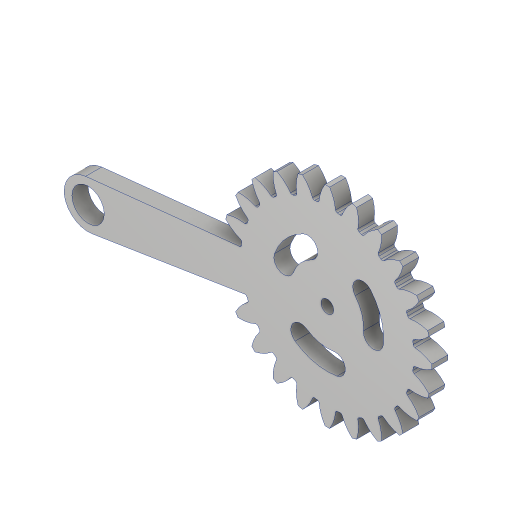
# Autodesk Inventor part: Gear(PCD 48, MOD 2)
Saved by Autodesk Inventor 2023.2 (Build 272271000, 271)
## iProperties
Created: 2021-07-28
Part Number: Gear(PCD 48, MOD 2)
Material: 알루미늄 6061
Document SubType Name: Modeling
Designer: user
Density: 2.7 g/cm^3
Appearance: 알루미늄 - 평지
Mass: 26.9214 g
Surface Area: 65.457 cm^2
Volume: 9.97089 cm^3
Author: user
Autodesk Inventor part; units mm, degrees
(part 1 of 2)
ref_plane "YZ Plane" through (0, 0, 0) normal (1, 0, 0) x (0, 1, 0)
ref_plane "XZ Plane" through (0, 0, 0) normal (0, 1, 0) x (-1, 0, 0)
ref_plane "XY Plane" through (0, 0, 0) normal (0, 0, 1) x (1, 0, 0)
sketch "스케치1" plane through (0, 0, 0) normal (0, 0, 1) x (1, 0, 0)
  arc A0 (1.57, 23.9486) -> (-1.57, 23.9486) centre (0, 0) ccw
  arc A1 (-2.07, 21.4001) -> (2.07, 21.4001) centre (0, 0) ccw
  line L0 (0, 0) -> (0, 26)
  line L1 (-1.57, 0) -> (-1.57, 23.9486)
  line L2 (-0.57, 0) -> (-0.57, 25.9938)
  line L3 (-2.07, 0) -> (-2.07, 21.4001)
  arc A2 (-0.57, 25.9938) -> (-2.07, 21.4001) centre (7.2779, 20.8894) ccw
  line L4 (1.57, 0) -> (1.57, 23.9486)
  line L5 (0.57, 0) -> (0.57, 25.9938)
  line L6 (2.07, 0) -> (2.07, 21.4001)
  arc A3 (2.07, 21.4001) -> (0.57, 25.9938) centre (-7.2779, 20.8894) ccw
  arc A4 (0.57, 25.9938) -> (-0.57, 25.9938) centre (0, 0) ccw
  point P0 (-1.57, 29)
  point P1 (-0.57, 29)
  point P2 (-2.07, 29)
  point P3 (1.57, 29)
  point P4 (0.57, 29)
  point P5 (2.07, 29)
  dimension "d0" = 48
  dimension "d2" = 43
  dimension "d3" = 1.57
  dimension "d4" = 1
  dimension "d7" = 0.5
  constraints: 14 end point, 13 point on circle, 9 symmetric about line, 5 centre point, 3 coincident, 3 parallel, 1 vertical, 1 other
  measures "d0" diameter of A0
  measures "d2" diameter of A1
  measures "d3" distance between parallel lines of L0 L1
  measures "d4" distance between parallel lines of L1 L2
  measures "d7" distance between parallel lines of L3 L1
extrude "돌출1" add sketch "스케치1" along normal blind 4
sketch "스케치11" plane through (0, 0, 4) normal (0, 0, 1) x (1, 0, 0)
  circle A0 centre (0, 0) radius 1.6 projected
  arc A1 (13.9479, -1.2066) -> (10.7334, 8.9886) centre (0, 0) ccw projected
  arc A2 (8.9665, -0.7757) -> (13.9479, -1.2066) centre (11.4572, -0.9911) ccw projected
  arc A3 (8.9665, -0.7757) -> (6.9, 5.7784) centre (0, 0) ccw projected
  arc A4 (10.7334, 8.9886) -> (6.9, 5.7784) centre (8.8167, 7.3835) ccw projected
  arc A5 (-8.0189, -11.476) -> (2.4176, -13.7897) centre (0, 0) ccw projected
  arc A6 (-5.155, -7.3774) -> (-8.0189, -11.476) centre (-6.5869, -9.4267) ccw projected
  arc A7 (-5.155, -7.3774) -> (1.5542, -8.8648) centre (0, 0) ccw projected
  arc A8 (2.4176, -13.7897) -> (1.5542, -8.8648) centre (1.9859, -11.3272) ccw projected
  arc A9 (-3.8115, 8.1531) -> (-8.4542, 3.0864) centre (0, 0) ccw projected
  arc A10 (-13.151, 4.8011) -> (-8.4542, 3.0864) centre (-10.8026, 3.9438) ccw projected
  arc A11 (-5.929, 12.6825) -> (-13.151, 4.8011) centre (0, 0) ccw projected
  arc A12 (-3.8115, 8.1531) -> (-5.929, 12.6825) centre (-4.8703, 10.4178) ccw projected
  circle A13 centre (-59.4867, -7.8316) radius 4.025 projected
  arc A14 (-60.1049, -2.02) -> (-65.4557, -8.4603) centre (-59.4744, -7.9868) ccw projected
  arc A15 (-65.4557, -8.4603) -> (-58.5717, -13.6038) centre (-59.507, -7.6772) ccw projected
  line L0 (-58.5717, -13.6038) -> (-20.5345, -7.6012) projected
  arc A16 (-19.9916, -7.9111) -> (-20.5345, -7.6012) centre (-20.4565, -8.0951) ccw projected
  arc A17 (-19.9916, -7.9111) -> (-19.7349, -8.5314) centre (0, 0) ccw projected
  arc A18 (-19.9027, -9.1363) -> (-19.7349, -8.5314) centre (-20.1938, -8.7298) ccw projected
  arc A19 (-19.9027, -9.1363) -> (-22.7962, -12.5032) centre (-14.4518, -16.7475) ccw projected
  arc A20 (-22.7962, -12.5032) -> (-22.2262, -13.4905) centre (0, 0) ccw projected
  arc A21 (-22.2262, -13.4905) -> (-17.8636, -12.6681) centre (-21.7297, -4.1418) ccw projected
  arc A22 (-17.2558, -12.8252) -> (-17.8636, -12.6681) centre (-17.6571, -13.1235) ccw projected
  arc A23 (-17.2558, -12.8252) -> (-16.8544, -13.3484) centre (0, 0) ccw projected
  arc A24 (-16.8599, -13.9762) -> (-16.8544, -13.3484) centre (-17.2463, -13.6589) ccw projected
  arc A25 (-16.8599, -13.9762) -> (-18.7834, -17.9773) centre (-9.6248, -19.9173) ccw projected
  arc A26 (-18.7834, -17.9773) -> (-17.9773, -18.7834) centre (0, 0) ccw projected
  arc A27 (-17.9773, -18.7834) -> (-13.9762, -16.8599) centre (-19.9173, -9.6248) ccw projected
  arc A28 (-13.3484, -16.8544) -> (-13.9762, -16.8599) centre (-13.6589, -17.2463) ccw projected
  arc A29 (-13.3484, -16.8544) -> (-12.8252, -17.2558) centre (0, 0) ccw projected
  arc A30 (-12.6681, -17.8636) -> (-12.8252, -17.2558) centre (-13.1235, -17.6571) ccw projected
  arc A31 (-12.6681, -17.8636) -> (-13.4905, -22.2262) centre (-4.1418, -21.7297) ccw projected
  arc A32 (-13.4905, -22.2262) -> (-12.5032, -22.7962) centre (0, 0) ccw projected
  arc A33 (-12.5032, -22.7962) -> (-9.1363, -19.9027) centre (-16.7475, -14.4518) ccw projected
  arc A34 (-8.5314, -19.7349) -> (-9.1363, -19.9027) centre (-8.7298, -20.1938) ccw projected
  arc A35 (-8.5314, -19.7349) -> (-7.9221, -19.9873) centre (0, 0) ccw projected
  arc A36 (-7.613, -20.5337) -> (-7.9221, -19.9873) centre (-8.1063, -20.4521) ccw projected
  arc A37 (-7.613, -20.5337) -> (-7.2783, -24.9605) centre (1.6233, -22.0613) ccw projected
  arc A38 (-7.2783, -24.9605) -> (-6.1771, -25.2556) centre (0, 0) ccw projected
  arc A39 (-6.1771, -25.2556) -> (-3.6738, -21.5892) centre (-12.4365, -18.2939) ccw projected
  arc A40 (-3.1329, -21.2705) -> (-3.6738, -21.5892) centre (-3.2058, -21.7652) ccw projected
  arc A41 (-3.1329, -21.2705) -> (-2.4791, -21.3566) centre (0, 0) ccw projected
  arc A42 (-2.0391, -21.8044) -> (-2.4791, -21.3566) centre (-2.5367, -21.8533) ccw projected
  arc A43 (-2.0391, -21.8044) -> (-0.57, -25.9938) centre (7.2779, -20.8894) ccw projected
  arc A44 (-0.57, -25.9938) -> (0.57, -25.9938) centre (0, 0) ccw projected
  arc A45 (0.57, -25.9938) -> (2.0391, -21.8044) centre (-7.2779, -20.8894) ccw projected
  arc A46 (2.4791, -21.3566) -> (2.0391, -21.8044) centre (2.5367, -21.8533) ccw projected
  arc A47 (2.4791, -21.3566) -> (3.1329, -21.2705) centre (0, 0) ccw projected
  arc A48 (3.6738, -21.5892) -> (3.1329, -21.2705) centre (3.2058, -21.7652) ccw projected
  arc A49 (3.6738, -21.5892) -> (6.1771, -25.2556) centre (12.4365, -18.2939) ccw projected
  arc A50 (6.1771, -25.2556) -> (7.2783, -24.9605) centre (0, 0) ccw projected
  arc A51 (7.2783, -24.9605) -> (7.613, -20.5337) centre (-1.6233, -22.0613) ccw projected
  arc A52 (7.9221, -19.9873) -> (7.613, -20.5337) centre (8.1063, -20.4521) ccw projected
  arc A53 (7.9221, -19.9873) -> (8.5314, -19.7349) centre (0, 0) ccw projected
  arc A54 (9.1363, -19.9027) -> (8.5314, -19.7349) centre (8.7298, -20.1938) ccw projected
  arc A55 (9.1363, -19.9027) -> (12.5032, -22.7962) centre (16.7475, -14.4518) ccw projected
  arc A56 (12.5032, -22.7962) -> (13.4905, -22.2262) centre (0, 0) ccw projected
  arc A57 (13.4905, -22.2262) -> (12.6681, -17.8636) centre (4.1418, -21.7297) ccw projected
  arc A58 (12.8252, -17.2558) -> (12.6681, -17.8636) centre (13.1235, -17.6571) ccw projected
  arc A59 (12.8252, -17.2558) -> (13.3484, -16.8544) centre (0, 0) ccw projected
  arc A60 (13.9762, -16.8599) -> (13.3484, -16.8544) centre (13.6589, -17.2463) ccw projected
  arc A61 (13.9762, -16.8599) -> (17.9773, -18.7834) centre (19.9173, -9.6248) ccw projected
  arc A62 (17.9773, -18.7834) -> (18.7834, -17.9773) centre (0, 0) ccw projected
  arc A63 (18.7834, -17.9773) -> (16.8599, -13.9762) centre (9.6248, -19.9173) ccw projected
  arc A64 (16.8544, -13.3484) -> (16.8599, -13.9762) centre (17.2463, -13.6589) ccw projected
  arc A65 (16.8544, -13.3484) -> (17.2558, -12.8252) centre (0, 0) ccw projected
  arc A66 (17.8636, -12.6681) -> (17.2558, -12.8252) centre (17.6571, -13.1235) ccw projected
  arc A67 (17.8636, -12.6681) -> (22.2262, -13.4905) centre (21.7297, -4.1418) ccw projected
  arc A68 (22.2262, -13.4905) -> (22.7962, -12.5032) centre (0, 0) ccw projected
  arc A69 (22.7962, -12.5032) -> (19.9027, -9.1363) centre (14.4518, -16.7475) ccw projected
  arc A70 (19.7349, -8.5314) -> (19.9027, -9.1363) centre (20.1938, -8.7298) ccw projected
  arc A71 (19.7349, -8.5314) -> (19.9873, -7.9221) centre (0, 0) ccw projected
  arc A72 (20.5337, -7.613) -> (19.9873, -7.9221) centre (20.4521, -8.1063) ccw projected
  arc A73 (20.5337, -7.613) -> (24.9605, -7.2783) centre (22.0613, 1.6233) ccw projected
  arc A74 (24.9605, -7.2783) -> (25.2556, -6.1771) centre (0, 0) ccw projected
  arc A75 (25.2556, -6.1771) -> (21.5892, -3.6738) centre (18.2939, -12.4365) ccw projected
  arc A76 (21.2705, -3.1329) -> (21.5892, -3.6738) centre (21.7652, -3.2058) ccw projected
  arc A77 (21.2705, -3.1329) -> (21.3566, -2.4791) centre (0, 0) ccw projected
  arc A78 (21.8044, -2.0391) -> (21.3566, -2.4791) centre (21.8533, -2.5367) ccw projected
  arc A79 (21.8044, -2.0391) -> (25.9938, -0.57) centre (20.8894, 7.2779) ccw projected
  arc A80 (25.9938, -0.57) -> (25.9938, 0.57) centre (0, 0) ccw projected
  arc A81 (25.9938, 0.57) -> (21.8044, 2.0391) centre (20.8894, -7.2779) ccw projected
  arc A82 (21.3566, 2.4791) -> (21.8044, 2.0391) centre (21.8533, 2.5367) ccw projected
  arc A83 (21.3566, 2.4791) -> (21.2705, 3.1329) centre (0, 0) ccw projected
  arc A84 (21.5892, 3.6738) -> (21.2705, 3.1329) centre (21.7652, 3.2058) ccw projected
  arc A85 (21.5892, 3.6738) -> (25.2556, 6.1771) centre (18.2939, 12.4365) ccw projected
  arc A86 (25.2556, 6.1771) -> (24.9605, 7.2783) centre (0, 0) ccw projected
  arc A87 (24.9605, 7.2783) -> (20.5337, 7.613) centre (22.0613, -1.6233) ccw projected
  arc A88 (19.9873, 7.9221) -> (20.5337, 7.613) centre (20.4521, 8.1063) ccw projected
  arc A89 (19.9873, 7.9221) -> (19.7349, 8.5314) centre (0, 0) ccw projected
  arc A90 (19.9027, 9.1363) -> (19.7349, 8.5314) centre (20.1938, 8.7298) ccw projected
  arc A91 (19.9027, 9.1363) -> (22.7962, 12.5032) centre (14.4518, 16.7475) ccw projected
  arc A92 (22.7962, 12.5032) -> (22.2262, 13.4905) centre (0, 0) ccw projected
  arc A93 (22.2262, 13.4905) -> (17.8636, 12.6681) centre (21.7297, 4.1418) ccw projected
  arc A94 (17.2558, 12.8252) -> (17.8636, 12.6681) centre (17.6571, 13.1235) ccw projected
  arc A95 (17.2558, 12.8252) -> (16.8544, 13.3484) centre (0, 0) ccw projected
  arc A96 (16.8599, 13.9762) -> (16.8544, 13.3484) centre (17.2463, 13.6589) ccw projected
  arc A97 (16.8599, 13.9762) -> (18.7834, 17.9773) centre (9.6248, 19.9173) ccw projected
  arc A98 (18.7834, 17.9773) -> (17.9773, 18.7834) centre (0, 0) ccw projected
  arc A99 (17.9773, 18.7834) -> (13.9762, 16.8599) centre (19.9173, 9.6248) ccw projected
  arc A100 (13.3484, 16.8544) -> (13.9762, 16.8599) centre (13.6589, 17.2463) ccw projected
  arc A101 (13.3484, 16.8544) -> (12.8252, 17.2558) centre (0, 0) ccw projected
  arc A102 (12.6681, 17.8636) -> (12.8252, 17.2558) centre (13.1235, 17.6571) ccw projected
  arc A103 (12.6681, 17.8636) -> (13.4905, 22.2262) centre (4.1418, 21.7297) ccw projected
  arc A104 (13.4905, 22.2262) -> (12.5032, 22.7962) centre (0, 0) ccw projected
  arc A105 (12.5032, 22.7962) -> (9.1363, 19.9027) centre (16.7475, 14.4518) ccw projected
  arc A106 (8.5314, 19.7349) -> (9.1363, 19.9027) centre (8.7298, 20.1938) ccw projected
  arc A107 (8.5314, 19.7349) -> (7.9221, 19.9873) centre (0, 0) ccw projected
  arc A108 (7.613, 20.5337) -> (7.9221, 19.9873) centre (8.1063, 20.4521) ccw projected
  arc A109 (7.613, 20.5337) -> (7.2783, 24.9605) centre (-1.6233, 22.0613) ccw projected
  arc A110 (7.2783, 24.9605) -> (6.1771, 25.2556) centre (0, 0) ccw projected
  arc A111 (6.1771, 25.2556) -> (3.6738, 21.5892) centre (12.4365, 18.2939) ccw projected
  arc A112 (3.1329, 21.2705) -> (3.6738, 21.5892) centre (3.2058, 21.7652) ccw projected
  arc A113 (3.1329, 21.2705) -> (2.4791, 21.3566) centre (0, 0) ccw projected
  arc A114 (2.0391, 21.8044) -> (2.4791, 21.3566) centre (2.5367, 21.8533) ccw projected
  arc A115 (2.0391, 21.8044) -> (0.57, 25.9938) centre (-7.2779, 20.8894) ccw projected
  arc A116 (0.57, 25.9938) -> (-0.57, 25.9938) centre (0, 0) ccw projected
  arc A117 (-0.57, 25.9938) -> (-2.0391, 21.8044) centre (7.2779, 20.8894) ccw projected
  arc A118 (-2.4791, 21.3566) -> (-2.0391, 21.8044) centre (-2.5367, 21.8533) ccw projected
  arc A119 (-2.4791, 21.3566) -> (-3.1329, 21.2705) centre (0, 0) ccw projected
  arc A120 (-3.6738, 21.5892) -> (-3.1329, 21.2705) centre (-3.2058, 21.7652) ccw projected
  arc A121 (-3.6738, 21.5892) -> (-6.1771, 25.2556) centre (-12.4365, 18.2939) ccw projected
  arc A122 (-6.1771, 25.2556) -> (-7.2783, 24.9605) centre (0, 0) ccw projected
  arc A123 (-7.2783, 24.9605) -> (-7.613, 20.5337) centre (1.6233, 22.0613) ccw projected
  arc A124 (-7.9221, 19.9873) -> (-7.613, 20.5337) centre (-8.1063, 20.4521) ccw projected
  arc A125 (-7.9221, 19.9873) -> (-8.5314, 19.7349) centre (0, 0) ccw projected
  arc A126 (-9.1363, 19.9027) -> (-8.5314, 19.7349) centre (-8.7298, 20.1938) ccw projected
  arc A127 (-9.1363, 19.9027) -> (-12.5032, 22.7962) centre (-16.7475, 14.4518) ccw projected
  arc A128 (-12.5032, 22.7962) -> (-13.4905, 22.2262) centre (0, 0) ccw projected
  arc A129 (-13.4905, 22.2262) -> (-12.6681, 17.8636) centre (-4.1418, 21.7297) ccw projected
  arc A130 (-12.8252, 17.2558) -> (-12.6681, 17.8636) centre (-13.1235, 17.6571) ccw projected
  arc A131 (-12.8252, 17.2558) -> (-13.3484, 16.8544) centre (0, 0) ccw projected
  arc A132 (-13.9762, 16.8599) -> (-13.3484, 16.8544) centre (-13.6589, 17.2463) ccw projected
  arc A133 (-13.9762, 16.8599) -> (-17.9773, 18.7834) centre (-19.9173, 9.6248) ccw projected
  arc A134 (-17.9773, 18.7834) -> (-18.7834, 17.9773) centre (0, 0) ccw projected
  arc A135 (-18.7834, 17.9773) -> (-16.8599, 13.9762) centre (-9.6248, 19.9173) ccw projected
  arc A136 (-16.8544, 13.3484) -> (-16.8599, 13.9762) centre (-17.2463, 13.6589) ccw projected
  arc A137 (-16.8544, 13.3484) -> (-17.2558, 12.8252) centre (0, 0) ccw projected
  arc A138 (-17.8636, 12.6681) -> (-17.2558, 12.8252) centre (-17.6571, 13.1235) ccw projected
  arc A139 (-17.8636, 12.6681) -> (-22.2262, 13.4905) centre (-21.7297, 4.1418) ccw projected
  arc A140 (-22.2262, 13.4905) -> (-22.7962, 12.5032) centre (0, 0) ccw projected
  arc A141 (-22.7962, 12.5032) -> (-19.9027, 9.1363) centre (-14.4518, 16.7475) ccw projected
  arc A142 (-19.7349, 8.5314) -> (-19.9027, 9.1363) centre (-20.1938, 8.7298) ccw projected
  arc A143 (-19.7349, 8.5314) -> (-19.9873, 7.9221) centre (0, 0) ccw projected
  arc A144 (-20.5337, 7.613) -> (-19.9873, 7.9221) centre (-20.4521, 8.1063) ccw projected
  arc A145 (-20.5337, 7.613) -> (-24.9605, 7.2783) centre (-22.0613, -1.6233) ccw projected
  arc A146 (-24.9605, 7.2783) -> (-25.2556, 6.1771) centre (0, 0) ccw projected
  arc A147 (-25.2556, 6.1771) -> (-21.5892, 3.6738) centre (-18.2939, 12.4365) ccw projected
  arc A148 (-21.2705, 3.1329) -> (-21.5892, 3.6738) centre (-21.7652, 3.2058) ccw projected
  arc A149 (-21.2705, 3.1329) -> (-21.358, 2.4674) centre (0, 0) ccw projected
  arc A150 (-21.8021, 2.0275) -> (-21.358, 2.4674) centre (-21.8546, 2.5248) ccw projected
  line L1 (-21.8021, 2.0275) -> (-60.1049, -2.02) projected
  circle A151 centre (0, 0) radius 1.6 projected
  circle A152 centre (0, 0) radius 1.6
  constraints: 1 centre point, 1 coincident
sketch "스케치7" plane through (0, 0, 4) normal (0, 0, 1) x (1, 0, 0)
  circle A0 centre (-59.4867, -7.8316) radius 4.025 projected
  circle A1 centre (-59.4867, -7.8316) radius 4.8
  point P0 (0, 0)
  dimension "d46" = 9.6
  constraints: 1 centre point, 1 coincident
  measures "d46" diameter of A1
sketch "스케치8" plane through (0, 0, 4) normal (0, 0, 1) x (1, 0, 0)
  circle A0 centre (-59.4867, -7.8316) radius 4.8 projected
  arc A1 (13.9479, -1.2066) -> (10.7334, 8.9886) centre (0, 0) ccw projected
  arc A2 (8.9665, -0.7757) -> (13.9479, -1.2066) centre (11.4572, -0.9911) ccw projected
  arc A3 (8.9665, -0.7757) -> (6.9, 5.7784) centre (0, 0) ccw projected
  arc A4 (10.7334, 8.9886) -> (6.9, 5.7784) centre (8.8167, 7.3835) ccw projected
  arc A5 (-8.0189, -11.476) -> (2.4176, -13.7897) centre (0, 0) ccw projected
  arc A6 (-5.155, -7.3774) -> (-8.0189, -11.476) centre (-6.5869, -9.4267) ccw projected
  arc A7 (-5.155, -7.3774) -> (1.5542, -8.8648) centre (0, 0) ccw projected
  arc A8 (2.4176, -13.7897) -> (1.5542, -8.8648) centre (1.9859, -11.3272) ccw projected
  arc A9 (-3.8115, 8.1531) -> (-8.4542, 3.0864) centre (0, 0) ccw projected
  arc A10 (-13.151, 4.8011) -> (-8.4542, 3.0864) centre (-10.8026, 3.9438) ccw projected
  arc A11 (-5.929, 12.6825) -> (-13.151, 4.8011) centre (0, 0) ccw projected
  arc A12 (-3.8115, 8.1531) -> (-5.929, 12.6825) centre (-4.8703, 10.4178) ccw projected
  arc A13 (-60.1049, -2.02) -> (-65.4557, -8.4603) centre (-59.4744, -7.9868) ccw projected
  arc A14 (-65.4557, -8.4603) -> (-58.5717, -13.6038) centre (-59.507, -7.6772) ccw projected
  line L0 (-58.5717, -13.6038) -> (-20.5345, -7.6012) projected
  arc A15 (-19.9916, -7.9111) -> (-20.5345, -7.6012) centre (-20.4565, -8.0951) ccw projected
  arc A16 (-19.9916, -7.9111) -> (-19.7349, -8.5314) centre (0, 0) ccw projected
  arc A17 (-19.9027, -9.1363) -> (-19.7349, -8.5314) centre (-20.1938, -8.7298) ccw projected
  arc A18 (-19.9027, -9.1363) -> (-22.7962, -12.5032) centre (-14.4518, -16.7475) ccw projected
  arc A19 (-22.7962, -12.5032) -> (-22.2262, -13.4905) centre (0, 0) ccw projected
  arc A20 (-22.2262, -13.4905) -> (-17.8636, -12.6681) centre (-21.7297, -4.1418) ccw projected
  arc A21 (-17.2558, -12.8252) -> (-17.8636, -12.6681) centre (-17.6571, -13.1235) ccw projected
  arc A22 (-17.2558, -12.8252) -> (-16.8544, -13.3484) centre (0, 0) ccw projected
  arc A23 (-16.8599, -13.9762) -> (-16.8544, -13.3484) centre (-17.2463, -13.6589) ccw projected
  arc A24 (-16.8599, -13.9762) -> (-18.7834, -17.9773) centre (-9.6248, -19.9173) ccw projected
  arc A25 (-18.7834, -17.9773) -> (-17.9773, -18.7834) centre (0, 0) ccw projected
  arc A26 (-17.9773, -18.7834) -> (-13.9762, -16.8599) centre (-19.9173, -9.6248) ccw projected
  arc A27 (-13.3484, -16.8544) -> (-13.9762, -16.8599) centre (-13.6589, -17.2463) ccw projected
  arc A28 (-13.3484, -16.8544) -> (-12.8252, -17.2558) centre (0, 0) ccw projected
  arc A29 (-12.6681, -17.8636) -> (-12.8252, -17.2558) centre (-13.1235, -17.6571) ccw projected
  arc A30 (-12.6681, -17.8636) -> (-13.4905, -22.2262) centre (-4.1418, -21.7297) ccw projected
  arc A31 (-13.4905, -22.2262) -> (-12.5032, -22.7962) centre (0, 0) ccw projected
  arc A32 (-12.5032, -22.7962) -> (-9.1363, -19.9027) centre (-16.7475, -14.4518) ccw projected
  arc A33 (-8.5314, -19.7349) -> (-9.1363, -19.9027) centre (-8.7298, -20.1938) ccw projected
  arc A34 (-8.5314, -19.7349) -> (-7.9221, -19.9873) centre (0, 0) ccw projected
  arc A35 (-7.613, -20.5337) -> (-7.9221, -19.9873) centre (-8.1063, -20.4521) ccw projected
  arc A36 (-7.613, -20.5337) -> (-7.2783, -24.9605) centre (1.6233, -22.0613) ccw projected
  arc A37 (-7.2783, -24.9605) -> (-6.1771, -25.2556) centre (0, 0) ccw projected
  arc A38 (-6.1771, -25.2556) -> (-3.6738, -21.5892) centre (-12.4365, -18.2939) ccw projected
  arc A39 (-3.1329, -21.2705) -> (-3.6738, -21.5892) centre (-3.2058, -21.7652) ccw projected
  arc A40 (-3.1329, -21.2705) -> (-2.4791, -21.3566) centre (0, 0) ccw projected
  arc A41 (-2.0391, -21.8044) -> (-2.4791, -21.3566) centre (-2.5367, -21.8533) ccw projected
  arc A42 (-2.0391, -21.8044) -> (-0.57, -25.9938) centre (7.2779, -20.8894) ccw projected
  arc A43 (-0.57, -25.9938) -> (0.57, -25.9938) centre (0, 0) ccw projected
  arc A44 (0.57, -25.9938) -> (2.0391, -21.8044) centre (-7.2779, -20.8894) ccw projected
  arc A45 (2.4791, -21.3566) -> (2.0391, -21.8044) centre (2.5367, -21.8533) ccw projected
  arc A46 (2.4791, -21.3566) -> (3.1329, -21.2705) centre (0, 0) ccw projected
  arc A47 (3.6738, -21.5892) -> (3.1329, -21.2705) centre (3.2058, -21.7652) ccw projected
  arc A48 (3.6738, -21.5892) -> (6.1771, -25.2556) centre (12.4365, -18.2939) ccw projected
  arc A49 (6.1771, -25.2556) -> (7.2783, -24.9605) centre (0, 0) ccw projected
  arc A50 (7.2783, -24.9605) -> (7.613, -20.5337) centre (-1.6233, -22.0613) ccw projected
  arc A51 (7.9221, -19.9873) -> (7.613, -20.5337) centre (8.1063, -20.4521) ccw projected
  arc A52 (7.9221, -19.9873) -> (8.5314, -19.7349) centre (0, 0) ccw projected
  arc A53 (9.1363, -19.9027) -> (8.5314, -19.7349) centre (8.7298, -20.1938) ccw projected
  arc A54 (9.1363, -19.9027) -> (12.5032, -22.7962) centre (16.7475, -14.4518) ccw projected
  arc A55 (12.5032, -22.7962) -> (13.4905, -22.2262) centre (0, 0) ccw projected
  arc A56 (13.4905, -22.2262) -> (12.6681, -17.8636) centre (4.1418, -21.7297) ccw projected
  arc A57 (12.8252, -17.2558) -> (12.6681, -17.8636) centre (13.1235, -17.6571) ccw projected
  arc A58 (12.8252, -17.2558) -> (13.3484, -16.8544) centre (0, 0) ccw projected
  arc A59 (13.9762, -16.8599) -> (13.3484, -16.8544) centre (13.6589, -17.2463) ccw projected
  arc A60 (13.9762, -16.8599) -> (17.9773, -18.7834) centre (19.9173, -9.6248) ccw projected
  arc A61 (17.9773, -18.7834) -> (18.7834, -17.9773) centre (0, 0) ccw projected
  arc A62 (18.7834, -17.9773) -> (16.8599, -13.9762) centre (9.6248, -19.9173) ccw projected
  arc A63 (16.8544, -13.3484) -> (16.8599, -13.9762) centre (17.2463, -13.6589) ccw projected
  arc A64 (16.8544, -13.3484) -> (17.2558, -12.8252) centre (0, 0) ccw projected
  arc A65 (17.8636, -12.6681) -> (17.2558, -12.8252) centre (17.6571, -13.1235) ccw projected
  arc A66 (17.8636, -12.6681) -> (22.2262, -13.4905) centre (21.7297, -4.1418) ccw projected
  arc A67 (22.2262, -13.4905) -> (22.7962, -12.5032) centre (0, 0) ccw projected
  arc A68 (22.7962, -12.5032) -> (19.9027, -9.1363) centre (14.4518, -16.7475) ccw projected
  arc A69 (19.7349, -8.5314) -> (19.9027, -9.1363) centre (20.1938, -8.7298) ccw projected
  arc A70 (19.7349, -8.5314) -> (19.9873, -7.9221) centre (0, 0) ccw projected
  arc A71 (20.5337, -7.613) -> (19.9873, -7.9221) centre (20.4521, -8.1063) ccw projected
  arc A72 (20.5337, -7.613) -> (24.9605, -7.2783) centre (22.0613, 1.6233) ccw projected
  arc A73 (24.9605, -7.2783) -> (25.2556, -6.1771) centre (0, 0) ccw projected
  arc A74 (25.2556, -6.1771) -> (21.5892, -3.6738) centre (18.2939, -12.4365) ccw projected
  arc A75 (21.2705, -3.1329) -> (21.5892, -3.6738) centre (21.7652, -3.2058) ccw projected
  arc A76 (21.2705, -3.1329) -> (21.3566, -2.4791) centre (0, 0) ccw projected
  arc A77 (21.8044, -2.0391) -> (21.3566, -2.4791) centre (21.8533, -2.5367) ccw projected
  arc A78 (21.8044, -2.0391) -> (25.9938, -0.57) centre (20.8894, 7.2779) ccw projected
  arc A79 (25.9938, -0.57) -> (25.9938, 0.57) centre (0, 0) ccw projected
  arc A80 (25.9938, 0.57) -> (21.8044, 2.0391) centre (20.8894, -7.2779) ccw projected
  arc A81 (21.3566, 2.4791) -> (21.8044, 2.0391) centre (21.8533, 2.5367) ccw projected
  arc A82 (21.3566, 2.4791) -> (21.2705, 3.1329) centre (0, 0) ccw projected
  arc A83 (21.5892, 3.6738) -> (21.2705, 3.1329) centre (21.7652, 3.2058) ccw projected
  arc A84 (21.5892, 3.6738) -> (25.2556, 6.1771) centre (18.2939, 12.4365) ccw projected
  arc A85 (25.2556, 6.1771) -> (24.9605, 7.2783) centre (0, 0) ccw projected
  arc A86 (24.9605, 7.2783) -> (20.5337, 7.613) centre (22.0613, -1.6233) ccw projected
  arc A87 (19.9873, 7.9221) -> (20.5337, 7.613) centre (20.4521, 8.1063) ccw projected
  arc A88 (19.9873, 7.9221) -> (19.7349, 8.5314) centre (0, 0) ccw projected
  arc A89 (19.9027, 9.1363) -> (19.7349, 8.5314) centre (20.1938, 8.7298) ccw projected
  arc A90 (19.9027, 9.1363) -> (22.7962, 12.5032) centre (14.4518, 16.7475) ccw projected
  arc A91 (22.7962, 12.5032) -> (22.2262, 13.4905) centre (0, 0) ccw projected
  arc A92 (22.2262, 13.4905) -> (17.8636, 12.6681) centre (21.7297, 4.1418) ccw projected
  arc A93 (17.2558, 12.8252) -> (17.8636, 12.6681) centre (17.6571, 13.1235) ccw projected
  arc A94 (17.2558, 12.8252) -> (16.8544, 13.3484) centre (0, 0) ccw projected
  arc A95 (16.8599, 13.9762) -> (16.8544, 13.3484) centre (17.2463, 13.6589) ccw projected
  arc A96 (16.8599, 13.9762) -> (18.7834, 17.9773) centre (9.6248, 19.9173) ccw projected
  arc A97 (18.7834, 17.9773) -> (17.9773, 18.7834) centre (0, 0) ccw projected
  arc A98 (17.9773, 18.7834) -> (13.9762, 16.8599) centre (19.9173, 9.6248) ccw projected
  arc A99 (13.3484, 16.8544) -> (13.9762, 16.8599) centre (13.6589, 17.2463) ccw projected
  arc A100 (13.3484, 16.8544) -> (12.8252, 17.2558) centre (0, 0) ccw projected
  arc A101 (12.6681, 17.8636) -> (12.8252, 17.2558) centre (13.1235, 17.6571) ccw projected
  arc A102 (12.6681, 17.8636) -> (13.4905, 22.2262) centre (4.1418, 21.7297) ccw projected
  arc A103 (13.4905, 22.2262) -> (12.5032, 22.7962) centre (0, 0) ccw projected
  arc A104 (12.5032, 22.7962) -> (9.1363, 19.9027) centre (16.7475, 14.4518) ccw projected
  arc A105 (8.5314, 19.7349) -> (9.1363, 19.9027) centre (8.7298, 20.1938) ccw projected
  arc A106 (8.5314, 19.7349) -> (7.9221, 19.9873) centre (0, 0) ccw projected
  arc A107 (7.613, 20.5337) -> (7.9221, 19.9873) centre (8.1063, 20.4521) ccw projected
  arc A108 (7.613, 20.5337) -> (7.2783, 24.9605) centre (-1.6233, 22.0613) ccw projected
  arc A109 (7.2783, 24.9605) -> (6.1771, 25.2556) centre (0, 0) ccw projected
  arc A110 (6.1771, 25.2556) -> (3.6738, 21.5892) centre (12.4365, 18.2939) ccw projected
  arc A111 (3.1329, 21.2705) -> (3.6738, 21.5892) centre (3.2058, 21.7652) ccw projected
  arc A112 (3.1329, 21.2705) -> (2.4791, 21.3566) centre (0, 0) ccw projected
  arc A113 (2.0391, 21.8044) -> (2.4791, 21.3566) centre (2.5367, 21.8533) ccw projected
  arc A114 (2.0391, 21.8044) -> (0.57, 25.9938) centre (-7.2779, 20.8894) ccw projected
  arc A115 (0.57, 25.9938) -> (-0.57, 25.9938) centre (0, 0) ccw projected
  arc A116 (-0.57, 25.9938) -> (-2.0391, 21.8044) centre (7.2779, 20.8894) ccw projected
  arc A117 (-2.4791, 21.3566) -> (-2.0391, 21.8044) centre (-2.5367, 21.8533) ccw projected
  arc A118 (-2.4791, 21.3566) -> (-3.1329, 21.2705) centre (0, 0) ccw projected
  arc A119 (-3.6738, 21.5892) -> (-3.1329, 21.2705) centre (-3.2058, 21.7652) ccw projected
  arc A120 (-3.6738, 21.5892) -> (-6.1771, 25.2556) centre (-12.4365, 18.2939) ccw projected
  arc A121 (-6.1771, 25.2556) -> (-7.2783, 24.9605) centre (0, 0) ccw projected
  arc A122 (-7.2783, 24.9605) -> (-7.613, 20.5337) centre (1.6233, 22.0613) ccw projected
  arc A123 (-7.9221, 19.9873) -> (-7.613, 20.5337) centre (-8.1063, 20.4521) ccw projected
  arc A124 (-7.9221, 19.9873) -> (-8.5314, 19.7349) centre (0, 0) ccw projected
  arc A125 (-9.1363, 19.9027) -> (-8.5314, 19.7349) centre (-8.7298, 20.1938) ccw projected
  arc A126 (-9.1363, 19.9027) -> (-12.5032, 22.7962) centre (-16.7475, 14.4518) ccw projected
  arc A127 (-12.5032, 22.7962) -> (-13.4905, 22.2262) centre (0, 0) ccw projected
  arc A128 (-13.4905, 22.2262) -> (-12.6681, 17.8636) centre (-4.1418, 21.7297) ccw projected
  arc A129 (-12.8252, 17.2558) -> (-12.6681, 17.8636) centre (-13.1235, 17.6571) ccw projected
  arc A130 (-12.8252, 17.2558) -> (-13.3484, 16.8544) centre (0, 0) ccw projected
  arc A131 (-13.9762, 16.8599) -> (-13.3484, 16.8544) centre (-13.6589, 17.2463) ccw projected
  arc A132 (-13.9762, 16.8599) -> (-17.9773, 18.7834) centre (-19.9173, 9.6248) ccw projected
  arc A133 (-17.9773, 18.7834) -> (-18.7834, 17.9773) centre (0, 0) ccw projected
  arc A134 (-18.7834, 17.9773) -> (-16.8599, 13.9762) centre (-9.6248, 19.9173) ccw projected
  arc A135 (-16.8544, 13.3484) -> (-16.8599, 13.9762) centre (-17.2463, 13.6589) ccw projected
  arc A136 (-16.8544, 13.3484) -> (-17.2558, 12.8252) centre (0, 0) ccw projected
  arc A137 (-17.8636, 12.6681) -> (-17.2558, 12.8252) centre (-17.6571, 13.1235) ccw projected
  arc A138 (-17.8636, 12.6681) -> (-22.2262, 13.4905) centre (-21.7297, 4.1418) ccw projected
  arc A139 (-22.2262, 13.4905) -> (-22.7962, 12.5032) centre (0, 0) ccw projected
  arc A140 (-22.7962, 12.5032) -> (-19.9027, 9.1363) centre (-14.4518, 16.7475) ccw projected
  arc A141 (-19.7349, 8.5314) -> (-19.9027, 9.1363) centre (-20.1938, 8.7298) ccw projected
  arc A142 (-19.7349, 8.5314) -> (-19.9873, 7.9221) centre (0, 0) ccw projected
  arc A143 (-20.5337, 7.613) -> (-19.9873, 7.9221) centre (-20.4521, 8.1063) ccw projected
  arc A144 (-20.5337, 7.613) -> (-24.9605, 7.2783) centre (-22.0613, -1.6233) ccw projected
  arc A145 (-24.9605, 7.2783) -> (-25.2556, 6.1771) centre (0, 0) ccw projected
  arc A146 (-25.2556, 6.1771) -> (-21.5892, 3.6738) centre (-18.2939, 12.4365) ccw projected
  arc A147 (-21.2705, 3.1329) -> (-21.5892, 3.6738) centre (-21.7652, 3.2058) ccw projected
  arc A148 (-21.2705, 3.1329) -> (-21.358, 2.4674) centre (0, 0) ccw projected
  arc A149 (-21.8021, 2.0275) -> (-21.358, 2.4674) centre (-21.8546, 2.5248) ccw projected
  line L1 (-21.8021, 2.0275) -> (-60.1049, -2.02) projected
  circle A150 centre (0, 0) radius 3.5 projected
  circle A151 centre (0, 0) radius 1.25 projected
  circle A152 centre (0, 0) radius 3.5 projected
pattern_circular "원형 패턴1" count 24 over 360 about axis through (0, 0, 0) along (0, 0, 1) of "돌출1"
sketch "스케치2" plane through (0, 0, 4) normal (0, 0, 1) x (1, 0, 0)
  circle A0 centre (0, 0) radius 3.5
  dimension "d13" = 7
  constraints: 1 centre point, 1 coincident
  measures "d13" diameter of A0
extrude "돌출2" add sketch "스케치2" along normal blind 3
sketch "스케치3" plane through (0, 0, 7) normal (0, 0, 1) x (1, 0, 0)
  circle A0 centre (0, 0) radius 1.25
  dimension "d16" = 2.5
  constraints: 1 centre point, 1 coincident
  measures "d16" diameter of A0
extrude "돌출3" cut sketch "스케치3" against normal up to surface (7 mm away)
sketch "스케치4" plane through (0, 0, 4) normal (0, 0, 1) x (1, 0, 0)
  circle A0 centre (0, 0) radius 21.5
  arc A1 (-25.9938, -0.57) -> (-21.4001, -2.07) centre (-20.8894, 7.2779) ccw projected
  arc A2 (-25.9938, 0.57) -> (-25.9938, -0.57) centre (0, 0) ccw projected
  arc A3 (-21.4001, 2.07) -> (-25.9938, 0.57) centre (-20.8894, -7.2779) ccw projected
  arc A4 (-21.2067, -3.5393) -> (-25.2556, -6.1771) centre (-18.2939, -12.4365) ccw projected
  arc A5 (-25.2556, -6.1771) -> (-24.9605, -7.2783) centre (0, 0) ccw projected
  arc A6 (-24.9605, -7.2783) -> (-20.1352, -7.5382) centre (-22.0613, 1.6233) ccw projected
  dimension "d19" = 43
  constraints: 1 centre point, 1 coincident
  measures "d19" diameter of A0
extrude "돌출4" cut sketch "스케치4" against normal up to surface (4 mm away) contours A0 A1 A2 A3 | A6 A5 A4 A0
sketch "스케치5" plane through (0, 0, 4) normal (0, 0, 1) x (1, 0, 0)
  line L0 (0, 0) -> (21.3161, 2.8063)
  arc A0 (21.4001, 2.07) -> (21.2067, 3.5393) centre (0, 0) ccw projected
  line L1 (0, 0) -> (21.5, 0) construction
  line L2 (0, 0) -> (-21.3161, -2.8063)
  arc A1 (-21.2067, 3.5393) -> (-19.568, -8.9074) centre (0, 0) ccw projected
  line L3 (0, 0) -> (-65.4354, -8.6147)
  line L4 (0, 0) -> (66, 0) construction
  line L5 (-65.4354, -8.6147) -> (-64.6522, -14.5634)
  line L6 (-65.4354, -8.6147) -> (-66.2185, -2.6661)
  arc A2 (-20.1352, -7.5382) -> (-19.568, -8.9074) centre (0, 0) ccw projected
  line L7 (-64.6522, -14.5634) -> (-20.1352, -7.5382)
  arc A3 (-21.2067, 3.5393) -> (-21.4001, 2.07) centre (0, 0) ccw projected
  line L8 (-66.2185, -2.6661) -> (-21.4001, 2.07)
  line L9 (0, 0) -> (-59.4867, -7.8316)
  line L10 (0, 0) -> (60, 0) construction
  circle A4 centre (-59.4867, -7.8316) radius 4.025
  dimension "d22" = 7.5
  dimension "d23" = 66
  dimension "d24" = 172.5
  dimension "d25" = 6
  dimension "d26" = 90
  dimension "d27" = 6
  dimension "d28" = 60
  dimension "d29" = 172.5
  dimension "d30" = 8.05
  constraints: 22 end point, 3 collinear, 3 equal length, 3 horizontal, 2 point on circle, 1 centre point, 1 coincident, 1 perpendicular
  measures "d22" angle of L1 L0
  measures "d23" distance of L3.start L3.end
  measures "d24" angle of L3 L4
  measures "d25" distance of L3.end L5.end
  measures "d26" angle of L5 L3
  measures "d27" distance of L3.end L6.end
  measures "d28" distance of L9.start L9.end
  measures "d29" angle of L9 L10
  measures "d30" diameter of A4
extrude "돌출5" add sketch "스케치5" against normal up to surface (4 mm away) contours A1 L3 A4 L6 L8 | A1 L7 L5 L3 A4
fillet "모깎기1" radius 6 2 edges at (-64.6522, -14.5634, 2) (-66.2185, -2.6661, 2)
fillet "모깎기2" radius 0.5 46 edges at (-21.4001, 2.07, 2) (-20.1352, 7.5382, 2) (-19.568, 8.9074, 2) (-21.2067, 3.5393, 2) (-17.498, 12.4927, 2) (-16.5959, 13.6685, 2) (-12.4927, 17.498, 2) (-7.5382, 20.1352, 2) (-2.07, 21.4001, 2) (3.5393, 21.2067, 2) (8.9074, 19.568, 2) (-13.6685, 16.5959, 2) (-8.9074, 19.568, 2) (-3.5393, 21.2067, 2) (2.07, 21.4001, 2) (7.5382, 20.1352, 2) (12.4927, 17.498, 2) (13.6685, 16.5959, 2) (17.498, 12.4927, 2) (16.5959, 13.6685, 2) (19.568, 8.9074, 2) (20.1352, 7.5382, 2) (21.4001, 2.07, 2) (21.2067, 3.5393, 2) (21.4001, -2.07, 2) (21.2067, -3.5393, 2) (19.568, -8.9074, 2) (20.1352, -7.5382, 2) (16.5959, -13.6685, 2) (12.4927, -17.498, 2) (17.498, -12.4927, 2) (13.6685, -16.5959, 2) (7.5382, -20.1352, 2) (2.07, -21.4001, 2) (8.9074, -19.568, 2) (3.5393, -21.2067, 2) (-3.5393, -21.2067, 2) (-8.9074, -19.568, 2) (-13.6685, -16.5959, 2) (-17.498, -12.4927, 2) (-2.07, -21.4001, 2) (-7.5382, -20.1352, 2) (-12.4927, -17.498, 2) (-16.5959, -13.6685, 2) (-19.568, -8.9074, 2) (-20.1352, -7.5382, 2)
sketch "스케치6" plane through (0, 0, 0) normal (0, 0, -1) x (-1, 0, 0)
  arc A0 (9, 0) -> (6.6355, -6.0803) centre (0, 0) ccw
  arc A1 (14, 0) -> (10.3219, -9.4583) centre (0, 0) ccw
  circle A2 centre (0, 0) radius 1.25 projected
  line L0 (0, 0) -> (14, 0) construction
  line L1 (0, 0) -> (14, 0) construction
  line L2 (0, 0) -> (14, 0) construction
  line L3 (0, 0) -> (14, 0) construction
  line L4 (0, 0) -> (14, 0) construction
  line L5 (0, 0) -> (14, 0) construction
  line L6 (0, 0) -> (1.2393, 0.1632)
  line L7 (8.923, 1.1747) -> (13.8802, 1.8274)
  line L8 (0, 0) -> (0.9216, -0.8445)
  line L9 (6.6355, -6.0803) -> (10.3219, -9.4583)
  line L10 (0, 0) -> (-0.4784, -1.1548)
  line L11 (-3.4442, -8.3149) -> (-5.3576, -12.9343)
  line L12 (0, 0) -> (-1.1921, -0.3759)
  line L13 (-8.5835, -2.7064) -> (-13.352, -4.2099)
  line L14 (0, 0) -> (-0.761, 0.9917)
  line L15 (-5.4789, 7.1402) -> (-8.5227, 11.1069)
  line L16 (0, 0) -> (0.2705, 1.2204)
  line L17 (1.948, 8.7867) -> (3.0302, 13.6681)
  dimension "d35" = 18
  dimension "d36" = 28
  constraints: 36 end point, 20 point on circle, 6 horizontal, 2 centre point, 2 coincident, 1 point on line
  measures "d35" diameter of A0
  measures "d36" diameter of A1
extrude "돌출6" cut sketch "스케치6" against normal up to surface (4 mm away) contours A0 L17 A1 L7 | A0 L13 A1 L15 | A0 L9 A1 L11
fillet "모깎기3" radius 2.5 12 edges at (5.3576, -12.9343, 2) (3.4442, -8.3149, 2) (-10.3219, -9.4583, 2) (-6.6355, -6.0803, 2) (-8.923, 1.1747, 2) (-1.948, 8.7867, 2) (-3.0302, 13.6681, 2) (-13.8802, 1.8274, 2) (8.5835, -2.7064, 2) (5.4789, 7.1402, 2) (13.352, -4.2099, 2) (8.5227, 11.1069, 2)
sketch "스케치9" plane through (0, 0, 4) normal (0, 0, 1) x (1, 0, 0)
  arc A0 (13.9479, -1.2066) -> (10.7334, 8.9886) centre (0, 0) ccw projected
  arc A1 (8.9665, -0.7757) -> (13.9479, -1.2066) centre (11.4572, -0.9911) ccw projected
  arc A2 (8.9665, -0.7757) -> (6.9, 5.7784) centre (0, 0) ccw projected
  arc A3 (10.7334, 8.9886) -> (6.9, 5.7784) centre (8.8167, 7.3835) ccw projected
  arc A4 (-8.0189, -11.476) -> (2.4176, -13.7897) centre (0, 0) ccw projected
  arc A5 (-5.155, -7.3774) -> (-8.0189, -11.476) centre (-6.5869, -9.4267) ccw projected
  arc A6 (-5.155, -7.3774) -> (1.5542, -8.8648) centre (0, 0) ccw projected
  arc A7 (2.4176, -13.7897) -> (1.5542, -8.8648) centre (1.9859, -11.3272) ccw projected
  arc A8 (-3.8115, 8.1531) -> (-8.4542, 3.0864) centre (0, 0) ccw projected
  arc A9 (-13.151, 4.8011) -> (-8.4542, 3.0864) centre (-10.8026, 3.9438) ccw projected
  arc A10 (-5.929, 12.6825) -> (-13.151, 4.8011) centre (0, 0) ccw projected
  arc A11 (-3.8115, 8.1531) -> (-5.929, 12.6825) centre (-4.8703, 10.4178) ccw projected
  circle A12 centre (-59.4867, -7.8316) radius 4.025 projected
  arc A13 (-60.1049, -2.02) -> (-65.4557, -8.4603) centre (-59.4744, -7.9868) ccw projected
  arc A14 (-65.4557, -8.4603) -> (-58.5717, -13.6038) centre (-59.507, -7.6772) ccw projected
  line L0 (-58.5717, -13.6038) -> (-20.5345, -7.6012) projected
  arc A15 (-19.9916, -7.9111) -> (-20.5345, -7.6012) centre (-20.4565, -8.0951) ccw projected
  arc A16 (-19.9916, -7.9111) -> (-19.7349, -8.5314) centre (0, 0) ccw projected
  arc A17 (-19.9027, -9.1363) -> (-19.7349, -8.5314) centre (-20.1938, -8.7298) ccw projected
  arc A18 (-19.9027, -9.1363) -> (-22.7962, -12.5032) centre (-14.4518, -16.7475) ccw projected
  arc A19 (-22.7962, -12.5032) -> (-22.2262, -13.4905) centre (0, 0) ccw projected
  arc A20 (-22.2262, -13.4905) -> (-17.8636, -12.6681) centre (-21.7297, -4.1418) ccw projected
  arc A21 (-17.2558, -12.8252) -> (-17.8636, -12.6681) centre (-17.6571, -13.1235) ccw projected
  arc A22 (-17.2558, -12.8252) -> (-16.8544, -13.3484) centre (0, 0) ccw projected
  arc A23 (-16.8599, -13.9762) -> (-16.8544, -13.3484) centre (-17.2463, -13.6589) ccw projected
  arc A24 (-16.8599, -13.9762) -> (-18.7834, -17.9773) centre (-9.6248, -19.9173) ccw projected
  arc A25 (-18.7834, -17.9773) -> (-17.9773, -18.7834) centre (0, 0) ccw projected
  arc A26 (-17.9773, -18.7834) -> (-13.9762, -16.8599) centre (-19.9173, -9.6248) ccw projected
  arc A27 (-13.3484, -16.8544) -> (-13.9762, -16.8599) centre (-13.6589, -17.2463) ccw projected
  arc A28 (-13.3484, -16.8544) -> (-12.8252, -17.2558) centre (0, 0) ccw projected
  arc A29 (-12.6681, -17.8636) -> (-12.8252, -17.2558) centre (-13.1235, -17.6571) ccw projected
  arc A30 (-12.6681, -17.8636) -> (-13.4905, -22.2262) centre (-4.1418, -21.7297) ccw projected
  arc A31 (-13.4905, -22.2262) -> (-12.5032, -22.7962) centre (0, 0) ccw projected
  arc A32 (-12.5032, -22.7962) -> (-9.1363, -19.9027) centre (-16.7475, -14.4518) ccw projected
  arc A33 (-8.5314, -19.7349) -> (-9.1363, -19.9027) centre (-8.7298, -20.1938) ccw projected
  arc A34 (-8.5314, -19.7349) -> (-7.9221, -19.9873) centre (0, 0) ccw projected
  arc A35 (-7.613, -20.5337) -> (-7.9221, -19.9873) centre (-8.1063, -20.4521) ccw projected
  arc A36 (-7.613, -20.5337) -> (-7.2783, -24.9605) centre (1.6233, -22.0613) ccw projected
  arc A37 (-7.2783, -24.9605) -> (-6.1771, -25.2556) centre (0, 0) ccw projected
  arc A38 (-6.1771, -25.2556) -> (-3.6738, -21.5892) centre (-12.4365, -18.2939) ccw projected
  arc A39 (-3.1329, -21.2705) -> (-3.6738, -21.5892) centre (-3.2058, -21.7652) ccw projected
  arc A40 (-3.1329, -21.2705) -> (-2.4791, -21.3566) centre (0, 0) ccw projected
  arc A41 (-2.0391, -21.8044) -> (-2.4791, -21.3566) centre (-2.5367, -21.8533) ccw projected
  arc A42 (-2.0391, -21.8044) -> (-0.57, -25.9938) centre (7.2779, -20.8894) ccw projected
  arc A43 (-0.57, -25.9938) -> (0.57, -25.9938) centre (0, 0) ccw projected
  arc A44 (0.57, -25.9938) -> (2.0391, -21.8044) centre (-7.2779, -20.8894) ccw projected
  arc A45 (2.4791, -21.3566) -> (2.0391, -21.8044) centre (2.5367, -21.8533) ccw projected
  arc A46 (2.4791, -21.3566) -> (3.1329, -21.2705) centre (0, 0) ccw projected
  arc A47 (3.6738, -21.5892) -> (3.1329, -21.2705) centre (3.2058, -21.7652) ccw projected
  arc A48 (3.6738, -21.5892) -> (6.1771, -25.2556) centre (12.4365, -18.2939) ccw projected
  arc A49 (6.1771, -25.2556) -> (7.2783, -24.9605) centre (0, 0) ccw projected
  arc A50 (7.2783, -24.9605) -> (7.613, -20.5337) centre (-1.6233, -22.0613) ccw projected
  arc A51 (7.9221, -19.9873) -> (7.613, -20.5337) centre (8.1063, -20.4521) ccw projected
  arc A52 (7.9221, -19.9873) -> (8.5314, -19.7349) centre (0, 0) ccw projected
  arc A53 (9.1363, -19.9027) -> (8.5314, -19.7349) centre (8.7298, -20.1938) ccw projected
  arc A54 (9.1363, -19.9027) -> (12.5032, -22.7962) centre (16.7475, -14.4518) ccw projected
  arc A55 (12.5032, -22.7962) -> (13.4905, -22.2262) centre (0, 0) ccw projected
  arc A56 (13.4905, -22.2262) -> (12.6681, -17.8636) centre (4.1418, -21.7297) ccw projected
  arc A57 (12.8252, -17.2558) -> (12.6681, -17.8636) centre (13.1235, -17.6571) ccw projected
  arc A58 (12.8252, -17.2558) -> (13.3484, -16.8544) centre (0, 0) ccw projected
  arc A59 (13.9762, -16.8599) -> (13.3484, -16.8544) centre (13.6589, -17.2463) ccw projected
  arc A60 (13.9762, -16.8599) -> (17.9773, -18.7834) centre (19.9173, -9.6248) ccw projected
  arc A61 (17.9773, -18.7834) -> (18.7834, -17.9773) centre (0, 0) ccw projected
  arc A62 (18.7834, -17.9773) -> (16.8599, -13.9762) centre (9.6248, -19.9173) ccw projected
  arc A63 (16.8544, -13.3484) -> (16.8599, -13.9762) centre (17.2463, -13.6589) ccw projected
  arc A64 (16.8544, -13.3484) -> (17.2558, -12.8252) centre (0, 0) ccw projected
  arc A65 (17.8636, -12.6681) -> (17.2558, -12.8252) centre (17.6571, -13.1235) ccw projected
  arc A66 (17.8636, -12.6681) -> (22.2262, -13.4905) centre (21.7297, -4.1418) ccw projected
  arc A67 (22.2262, -13.4905) -> (22.7962, -12.5032) centre (0, 0) ccw projected
  arc A68 (22.7962, -12.5032) -> (19.9027, -9.1363) centre (14.4518, -16.7475) ccw projected
  arc A69 (19.7349, -8.5314) -> (19.9027, -9.1363) centre (20.1938, -8.7298) ccw projected
  arc A70 (19.7349, -8.5314) -> (19.9873, -7.9221) centre (0, 0) ccw projected
  arc A71 (20.5337, -7.613) -> (19.9873, -7.9221) centre (20.4521, -8.1063) ccw projected
  arc A72 (20.5337, -7.613) -> (24.9605, -7.2783) centre (22.0613, 1.6233) ccw projected
  arc A73 (24.9605, -7.2783) -> (25.2556, -6.1771) centre (0, 0) ccw projected
  arc A74 (25.2556, -6.1771) -> (21.5892, -3.6738) centre (18.2939, -12.4365) ccw projected
  arc A75 (21.2705, -3.1329) -> (21.5892, -3.6738) centre (21.7652, -3.2058) ccw projected
  arc A76 (21.2705, -3.1329) -> (21.3566, -2.4791) centre (0, 0) ccw projected
  arc A77 (21.8044, -2.0391) -> (21.3566, -2.4791) centre (21.8533, -2.5367) ccw projected
  arc A78 (21.8044, -2.0391) -> (25.9938, -0.57) centre (20.8894, 7.2779) ccw projected
  arc A79 (25.9938, -0.57) -> (25.9938, 0.57) centre (0, 0) ccw projected
  arc A80 (25.9938, 0.57) -> (21.8044, 2.0391) centre (20.8894, -7.2779) ccw projected
  arc A81 (21.3566, 2.4791) -> (21.8044, 2.0391) centre (21.8533, 2.5367) ccw projected
  arc A82 (21.3566, 2.4791) -> (21.2705, 3.1329) centre (0, 0) ccw projected
  arc A83 (21.5892, 3.6738) -> (21.2705, 3.1329) centre (21.7652, 3.2058) ccw projected
  arc A84 (21.5892, 3.6738) -> (25.2556, 6.1771) centre (18.2939, 12.4365) ccw projected
  arc A85 (25.2556, 6.1771) -> (24.9605, 7.2783) centre (0, 0) ccw projected
  arc A86 (24.9605, 7.2783) -> (20.5337, 7.613) centre (22.0613, -1.6233) ccw projected
  arc A87 (19.9873, 7.9221) -> (20.5337, 7.613) centre (20.4521, 8.1063) ccw projected
  arc A88 (19.9873, 7.9221) -> (19.7349, 8.5314) centre (0, 0) ccw projected
  arc A89 (19.9027, 9.1363) -> (19.7349, 8.5314) centre (20.1938, 8.7298) ccw projected
  arc A90 (19.9027, 9.1363) -> (22.7962, 12.5032) centre (14.4518, 16.7475) ccw projected
  arc A91 (22.7962, 12.5032) -> (22.2262, 13.4905) centre (0, 0) ccw projected
  arc A92 (22.2262, 13.4905) -> (17.8636, 12.6681) centre (21.7297, 4.1418) ccw projected
  arc A93 (17.2558, 12.8252) -> (17.8636, 12.6681) centre (17.6571, 13.1235) ccw projected
  arc A94 (17.2558, 12.8252) -> (16.8544, 13.3484) centre (0, 0) ccw projected
  arc A95 (16.8599, 13.9762) -> (16.8544, 13.3484) centre (17.2463, 13.6589) ccw projected
  arc A96 (16.8599, 13.9762) -> (18.7834, 17.9773) centre (9.6248, 19.9173) ccw projected
  arc A97 (18.7834, 17.9773) -> (17.9773, 18.7834) centre (0, 0) ccw projected
  arc A98 (17.9773, 18.7834) -> (13.9762, 16.8599) centre (19.9173, 9.6248) ccw projected
  arc A99 (13.3484, 16.8544) -> (13.9762, 16.8599) centre (13.6589, 17.2463) ccw projected
  arc A100 (13.3484, 16.8544) -> (12.8252, 17.2558) centre (0, 0) ccw projected
  arc A101 (12.6681, 17.8636) -> (12.8252, 17.2558) centre (13.1235, 17.6571) ccw projected
  arc A102 (12.6681, 17.8636) -> (13.4905, 22.2262) centre (4.1418, 21.7297) ccw projected
  arc A103 (13.4905, 22.2262) -> (12.5032, 22.7962) centre (0, 0) ccw projected
  arc A104 (12.5032, 22.7962) -> (9.1363, 19.9027) centre (16.7475, 14.4518) ccw projected
  arc A105 (8.5314, 19.7349) -> (9.1363, 19.9027) centre (8.7298, 20.1938) ccw projected
  arc A106 (8.5314, 19.7349) -> (7.9221, 19.9873) centre (0, 0) ccw projected
  arc A107 (7.613, 20.5337) -> (7.9221, 19.9873) centre (8.1063, 20.4521) ccw projected
  arc A108 (7.613, 20.5337) -> (7.2783, 24.9605) centre (-1.6233, 22.0613) ccw projected
  arc A109 (7.2783, 24.9605) -> (6.1771, 25.2556) centre (0, 0) ccw projected
  arc A110 (6.1771, 25.2556) -> (3.6738, 21.5892) centre (12.4365, 18.2939) ccw projected
  arc A111 (3.1329, 21.2705) -> (3.6738, 21.5892) centre (3.2058, 21.7652) ccw projected
  arc A112 (3.1329, 21.2705) -> (2.4791, 21.3566) centre (0, 0) ccw projected
  arc A113 (2.0391, 21.8044) -> (2.4791, 21.3566) centre (2.5367, 21.8533) ccw projected
  arc A114 (2.0391, 21.8044) -> (0.57, 25.9938) centre (-7.2779, 20.8894) ccw projected
  arc A115 (0.57, 25.9938) -> (-0.57, 25.9938) centre (0, 0) ccw projected
  arc A116 (-0.57, 25.9938) -> (-2.0391, 21.8044) centre (7.2779, 20.8894) ccw projected
  arc A117 (-2.4791, 21.3566) -> (-2.0391, 21.8044) centre (-2.5367, 21.8533) ccw projected
  arc A118 (-2.4791, 21.3566) -> (-3.1329, 21.2705) centre (0, 0) ccw projected
  arc A119 (-3.6738, 21.5892) -> (-3.1329, 21.2705) centre (-3.2058, 21.7652) ccw projected
  arc A120 (-3.6738, 21.5892) -> (-6.1771, 25.2556) centre (-12.4365, 18.2939) ccw projected
  arc A121 (-6.1771, 25.2556) -> (-7.2783, 24.9605) centre (0, 0) ccw projected
  arc A122 (-7.2783, 24.9605) -> (-7.613, 20.5337) centre (1.6233, 22.0613) ccw projected
  arc A123 (-7.9221, 19.9873) -> (-7.613, 20.5337) centre (-8.1063, 20.4521) ccw projected
  arc A124 (-7.9221, 19.9873) -> (-8.5314, 19.7349) centre (0, 0) ccw projected
  arc A125 (-9.1363, 19.9027) -> (-8.5314, 19.7349) centre (-8.7298, 20.1938) ccw projected
  arc A126 (-9.1363, 19.9027) -> (-12.5032, 22.7962) centre (-16.7475, 14.4518) ccw projected
  arc A127 (-12.5032, 22.7962) -> (-13.4905, 22.2262) centre (0, 0) ccw projected
  arc A128 (-13.4905, 22.2262) -> (-12.6681, 17.8636) centre (-4.1418, 21.7297) ccw projected
  arc A129 (-12.8252, 17.2558) -> (-12.6681, 17.8636) centre (-13.1235, 17.6571) ccw projected
  arc A130 (-12.8252, 17.2558) -> (-13.3484, 16.8544) centre (0, 0) ccw projected
  arc A131 (-13.9762, 16.8599) -> (-13.3484, 16.8544) centre (-13.6589, 17.2463) ccw projected
  arc A132 (-13.9762, 16.8599) -> (-17.9773, 18.7834) centre (-19.9173, 9.6248) ccw projected
  arc A133 (-17.9773, 18.7834) -> (-18.7834, 17.9773) centre (0, 0) ccw projected
  arc A134 (-18.7834, 17.9773) -> (-16.8599, 13.9762) centre (-9.6248, 19.9173) ccw projected
  arc A135 (-16.8544, 13.3484) -> (-16.8599, 13.9762) centre (-17.2463, 13.6589) ccw projected
  arc A136 (-16.8544, 13.3484) -> (-17.2558, 12.8252) centre (0, 0) ccw projected
  arc A137 (-17.8636, 12.6681) -> (-17.2558, 12.8252) centre (-17.6571, 13.1235) ccw projected
  arc A138 (-17.8636, 12.6681) -> (-22.2262, 13.4905) centre (-21.7297, 4.1418) ccw projected
  arc A139 (-22.2262, 13.4905) -> (-22.7962, 12.5032) centre (0, 0) ccw projected
  arc A140 (-22.7962, 12.5032) -> (-19.9027, 9.1363) centre (-14.4518, 16.7475) ccw projected
  arc A141 (-19.7349, 8.5314) -> (-19.9027, 9.1363) centre (-20.1938, 8.7298) ccw projected
  arc A142 (-19.7349, 8.5314) -> (-19.9873, 7.9221) centre (0, 0) ccw projected
  arc A143 (-20.5337, 7.613) -> (-19.9873, 7.9221) centre (-20.4521, 8.1063) ccw projected
  arc A144 (-20.5337, 7.613) -> (-24.9605, 7.2783) centre (-22.0613, -1.6233) ccw projected
  arc A145 (-24.9605, 7.2783) -> (-25.2556, 6.1771) centre (0, 0) ccw projected
  arc A146 (-25.2556, 6.1771) -> (-21.5892, 3.6738) centre (-18.2939, 12.4365) ccw projected
  arc A147 (-21.2705, 3.1329) -> (-21.5892, 3.6738) centre (-21.7652, 3.2058) ccw projected
  arc A148 (-21.2705, 3.1329) -> (-21.358, 2.4674) centre (0, 0) ccw projected
  arc A149 (-21.8021, 2.0275) -> (-21.358, 2.4674) centre (-21.8546, 2.5248) ccw projected
  line L1 (-21.8021, 2.0275) -> (-60.1049, -2.02) projected
  circle A150 centre (0, 0) radius 3.5 projected
  circle A151 centre (0, 0) radius 1.25 projected
  circle A152 centre (0, 0) radius 3.5 projected
extrude "돌출9" cut sketch "스케치9" along normal up to surface (3 mm away) contours A150